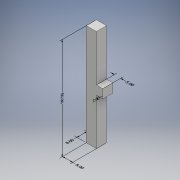
# Autodesk Inventor part: helicoptere
Saved by Autodesk Inventor 2018 (Build 220112000, 112)
## iProperties
Created: 2018-04-05
Part Number: helicoptere
Material: Générique
Document SubType Name: Modeling
Designer: Guadalix
Density: 1 g/cm^3
Appearance: Par défaut
Author: Guadalix
Autodesk Inventor part; units mm, degrees
ref_plane "YZ Plane" through (0, 0, 0) normal (1, 0, 0) x (0, 1, 0)
ref_plane "XZ Plane" through (0, 0, 0) normal (0, 1, 0) x (-1, 0, 0)
ref_plane "XY Plane" through (0, 0, 0) normal (0, 0, 1) x (1, 0, 0)
sketch "Esquisse1" plane through (0, 0, 0) normal (0, 1, 0) x (-1, 0, 0)
  line L0 (0, 0) -> (8, 0)
  line L1 (8, 0) -> (8, -40)
  line L2 (8, -40) -> (0, -40)
  line L3 (0, -40) -> (0, 0)
  line L4 (0, 0) -> (8, 0)
  line L5 (8, 0) -> (8, 40)
  line L6 (8, 40) -> (0, 40)
  line L7 (0, 40) -> (0, 0)
  line L8 (0, 3.5) -> (-5, 3.5)
  line L9 (-5, 3.5) -> (-5, 0)
  line L10 (-5, 0) -> (0, 0)
  line L11 (0, 0) -> (0, 3.5)
  line L12 (-5, -3.5) -> (0, -3.5)
  line L13 (0, -3.5) -> (0, 0)
  line L14 (0, 0) -> (-5, 0)
  line L15 (-5, 0) -> (-5, -3.5)
  dimension "d0" = 40
  dimension "d1" = 40
  dimension "d2" = 8
  dimension "d3" = 8
  dimension "d4" = 3.5
  dimension "d5" = 3.5
  dimension "d6" = 5
  dimension "d7" = 5
  constraints: 32 end point, 8 parallel, 4 horizontal, 4 perpendicular, 3 point on line
  measures "d0" distance of L0.end L1.end
  measures "d1" distance of L4.end L5.end
  measures "d2" distance of L5.end L6.end
  measures "d3" distance of L1.end L2.end
  measures "d4" distance of L8.end L9.end
  measures "d5" distance of L14.end L12.start
  measures "d6" distance of L12.start L12.end
  measures "d7" distance of L8.start L8.end
extrude "Extrusion1" add sketch "Esquisse1" along normal blind 8
sketch "Esquisse2" plane through (0, 8, 0) normal (0, 1, 0) x (1, 0, 0)
  line L0 (4.25, 2.5) -> (1.25, 2.5)
  line L1 (1.25, 2.5) -> (1.25, -2.5)
  line L2 (1.25, -2.5) -> (4.25, -2.5)
  line L3 (4.25, -2.5) -> (4.25, 2.5)
  line L4 (0, 0) -> (3, 0)
  line L5 (3, -10) -> (3, 10)
  line L6 (1.25, -2.5) -> (4.25, 2.5)
  line L7 (4.25, 2.5) -> (1.25, 2.5)
  line L8 (4.25, -2.5) -> (1.25, 2.5)
  line L9 (-8, 40) -> (-8, -40) projected
  line L10 (0, 3.5) -> (0, 40) projected
  line L11 (0, 40) -> (-8, 40) projected
  line L12 (0, 40) -> (-8, 40)
  line L13 (-5.5, -39.9859) -> (-4, 40)
  line L14 (0, 0) -> (-4.75, 0.007)
  point P0 (4.25, 0)
  point P1 (2.75, 0)
  dimension "d7" = 5
  dimension "d15" = 0
  dimension "d10" = 5
  dimension "d11" = 3
  dimension "d33" = 40
  dimension "d34" = 2.5
  dimension "d35" = 7.5
  constraints: 24 end point, 5 midpoint, 4 equal length, 2 coincident, 1 horizontal, 1 perpendicular, 1 other
  measures "d10" distance of L2.end L0.start
  measures "d11" distance of L1.end L2.end
  measures "d33" distance of L13.start L14.end
  measures "d34" distance of L9.end L13.start
  measures "d35" distance of L14.end point (2.75, 0)
extrude "Extrusion2" cut sketch "Esquisse2" against normal blind 7
fillet "Congé1" radius 0.1 1 edges at (1.25, 4.5, -2.5)
fillet "Congé2" radius 0.1 1 edges at (4.25, 4.5, -2.5)
fillet "Congé3" radius 0.1 1 edges at (4.25, 4.5, 2.5)
fillet "Congé4" radius 0.1 1 edges at (1.25, 4.5, 2.5)
